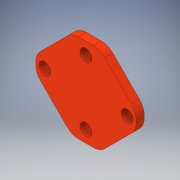
# Autodesk Inventor part: KugelradAdapter
Saved by Autodesk Inventor 2017 SP1 (Build 210196100, 196)
## iProperties
Part Number: KugelradAdapter
Material: Generisch
Document SubType Name: Modeling
Designer: Alex
Density: 1 g/cm^3
Appearance: Vorgabe
Author: Alex
Autodesk Inventor part; units mm, degrees
ref_plane "YZ Plane" through (0, 0, 0) normal (1, 0, 0) x (0, 1, 0)
ref_plane "XZ Plane" through (0, 0, 0) normal (0, 1, 0) x (-1, 0, 0)
ref_plane "XY Plane" through (0, 0, 0) normal (0, 0, 1) x (1, 0, 0)
sketch "Skizze1" plane through (0, 0, 0) normal (0, 1, 0) x (-1, 0, 0)
  line L0 (0, 0) -> (25, 0)
  line L1 (25, 0) -> (25, -22)
  line L2 (25, -22) -> (0, -22)
  line L3 (0, -22) -> (0, 0)
  dimension "d0" = 25
  dimension "d1" = 22
  constraints: 8 end point, 2 parallel, 1 horizontal, 1 perpendicular
  measures "d0" distance of L1.end L2.end
  measures "d1" distance of L0.end L1.end
extrude "Extrusion1" add sketch "Skizze1" along normal blind 2
chamfer "Fase1" distance 9 angle 45 4 edges at (0, 1, 0) (0, 1, -22) (-25, 1, -22) (-25, 1, 0)
fillet "Rundung1" radius 4 8 edges at (-25, 1, -13) (-25, 1, -9) (-16, 1, 0) (-9, 1, 0) (0, 1, -9) (0, 1, -13) (-9, 1, -22) (-16, 1, -22)
sketch "Skizze2" plane through (0, 2, 0) normal (0, 1, 0) x (1, 0, 0)
  line L0 (0, 10.6569) -> (0, 11.3431) projected
  line L1 (-14.3431, 0) -> (-10.6569, 0) projected
  point P0 (0, 0)
  point P1 (-2.25, 11)
  point P2 (-22.75, 11)
  dimension "d8" = 2.25
  dimension "d9" = 20.5
  dimension "d10" = 11
  constraints: 1 horizontal alignment
  measures "d8" distance from line of point (-2.25, 11) L0
  measures "d9" distance of point (-22.75, 11) point (-2.25, 11)
  measures "d10" distance from line of L1 point (-2.25, 11)
sketch "Skizze3" plane through (0, 2, 0) normal (0, 1, 0) x (1, 0, 0)
  line L0 (-14.3431, 0) -> (-10.6569, 0) projected
  line L1 (0, 10.6569) -> (0, 11.3431) projected
  point P0 (0, 0)
  point P1 (-12.5, 3)
  point P2 (-12.5, 19)
  dimension "d11" = 16
  dimension "d12" = 3
  dimension "d13" = 12.5
  constraints: 1 vertical alignment
  measures "d11" distance of point (-12.5, 19) point (-12.5, 3)
  measures "d12" distance from line of L0 point (-12.5, 3)
  measures "d13" distance from line of L1 point (-12.5, 3)
hole "Bohrung1" at (-12.5, 2, -3) at (-12.5, 2, -19) direction (0, -1, 0) diameter 3 depth 8 tip angle 118
hole "Bohrung2" at (-2.25, 2, -11) at (-22.75, 2, -11) direction (0, -1, 0) diameter 3 depth 8 tip angle 118
